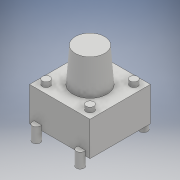
# Autodesk Inventor part: DTS-6-V
Saved by Autodesk Inventor 2017.3 (Build 213256000, 256)
## iProperties
Part Number: DTS-6-V
Material: 一般
Document SubType Name: Modeling
Designer: sktom
Density: 1 g/cm^3
Appearance: 既定
Author: sktom
Autodesk Inventor part; units mm, degrees
ref_plane "YZ Plane" through (0, 0, 0) normal (1, 0, 0) x (0, 1, 0)
ref_plane "XZ Plane" through (0, 0, 0) normal (0, 1, 0) x (-1, 0, 0)
ref_plane "XY Plane" through (0, 0, 0) normal (0, 0, 1) x (1, 0, 0)
sketch "スケッチ1" plane through (0, 0, 0) normal (0, 0, 1) x (1, 0, 0)
  line L0 (-3.1, -3.1) -> (3.1, -3.1)
  line L1 (3.1, -3.1) -> (3.1, 3.1)
  line L2 (3.1, 3.1) -> (-3.1, 3.1)
  line L3 (-3.1, 3.1) -> (-3.1, -3.1)
  line L4 (-3.1, -3.1) -> (3.1, 3.1) construction
  line L5 (3.1, -3.1) -> (-3.1, 3.1) construction
  point P0 (0, 0)
  dimension "d0" = 6.2
  dimension "d2" = 6.2
  constraints: 12 end point, 2 midpoint, 2 parallel, 1 horizontal, 1 perpendicular
  measures "d0" distance of L1.end L2.end
  measures "d2" distance of L0.end L1.end
extrude "押し出し1" add sketch "スケッチ1" along normal blind 3.5
sketch "スケッチ2" plane through (0, 0, 3.5) normal (0, 0, 1) x (1, 0, 0)
  line L0 (-2.25, -2.25) -> (2.25, -2.25) construction
  line L1 (2.25, -2.25) -> (2.25, 2.25) construction
  line L2 (2.25, 2.25) -> (-2.25, 2.25) construction
  line L3 (-2.25, 2.25) -> (-2.25, -2.25) construction
  line L4 (-2.25, -2.25) -> (2.25, 2.25) construction
  line L5 (2.25, -2.25) -> (-2.25, 2.25) construction
  circle A0 centre (-2.25, 2.25) radius 0.4
  circle A1 centre (2.25, 2.25) radius 0.4
  circle A2 centre (2.25, -2.25) radius 0.4
  circle A3 centre (-2.25, -2.25) radius 0.4
  point P0 (0, 0)
  dimension "d5" = 4.5
  dimension "d6" = 0.8
  constraints: 12 end point, 4 centre point, 4 coincident, 3 equal radius, 2 midpoint, 2 parallel, 2 perpendicular, 1 horizontal
  measures "d5" distance of L1.end L2.end
  measures "d6" diameter of A0
extrude "押し出し2" add sketch "スケッチ2" along normal blind 0.5
sketch "スケッチ3" plane through (0, 0, 0) normal (1, 0, 0) x (0, 1, 0)
  line L0 (3.1, 3.5) -> (-3.1, 3.5) projected
  line L1 (0, 3.5) -> (0, 7)
  line L2 (0, 7) -> (1.5, 7)
  line L3 (1.5, 7) -> (1.75, 3.5)
  line L4 (1.75, 3.5) -> (0, 3.5)
  point P0 (0, 0)
  dimension "d9" = 1.75
  dimension "d10" = 3.5
  dimension "d11" = 1.5
  constraints: 8 end point, 1 midpoint, 1 parallel, 1 perpendicular, 1 point on line, 1 vertical
  measures "d9" distance from line of L1 L3.end
  measures "d10" distance between parallel lines of L0 L2
  measures "d11" distance of L1.end L2.end
revolve "回転1" add sketch "スケッチ3" angle 360 about axis through (0, 0, 3.5) along (0, 0, 1)
sketch "スケッチ4" plane through (0, 0, 0) normal (0, 0, -1) x (-1, 0, 0)
  line L0 (2.25, -3.25) -> (-2.25, -3.25) construction
  line L1 (-2.25, -3.25) -> (-2.25, 3.25) construction
  line L2 (-2.25, 3.25) -> (2.25, 3.25) construction
  line L3 (2.25, 3.25) -> (2.25, -3.25) construction
  line L4 (2.25, -3.25) -> (-2.25, 3.25) construction
  line L5 (-2.25, -3.25) -> (2.25, 3.25) construction
  circle A0 centre (-2.25, 3.25) radius 0.4
  circle A1 centre (2.25, 3.25) radius 0.4
  circle A2 centre (2.25, -3.25) radius 0.4
  circle A3 centre (-2.25, -3.25) radius 0.4
  point P0 (0, 0)
  dimension "d13" = 4.5
  dimension "d14" = 6.5
  dimension "d15" = 0.8
  constraints: 12 end point, 4 centre point, 4 coincident, 3 equal radius, 2 midpoint, 2 parallel, 1 horizontal, 1 perpendicular
  measures "d13" distance of L1.end L2.end
  measures "d14" distance of L2.end L0.start
  measures "d15" diameter of A0
extrude "押し出し3" add sketch "スケッチ4" along normal blind 1 and the other way blind 0.5
